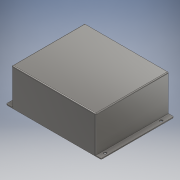
# Autodesk Inventor part: BatteryBox_NP1812
Saved by Autodesk Inventor 2018 (Build 220112000, 112)
## iProperties
Created: 2017-12-05
Part Number: BatteryBox_NP1812
Material: Steel, Galvanized
Document SubType Name: Modeling
Designer: P136265
Density: 7.85 g/cm^3
Appearance: Galvanized
Author: P136265
Autodesk Inventor part; units mm, degrees
ref_plane "YZ Plane" through (0, 0, 0) normal (1, 0, 0) x (0, 1, 0)
ref_plane "XZ Plane" through (0, 0, 0) normal (0, 1, 0) x (-1, 0, 0)
ref_plane "XY Plane" through (0, 0, 0) normal (0, 0, 1) x (1, 0, 0)
sketch "Sketch1" plane through (0, 0, 0) normal (0, 0, 1) x (1, 0, 0)
  line L0 (-92, -80) -> (92, -80)
  line L1 (92, -80) -> (92, 80)
  line L2 (92, 80) -> (-92, 80) construction
  line L3 (-92, 80) -> (-92, -80)
  line L4 (-92, -80) -> (92, 80) construction
  line L5 (92, -80) -> (-92, 80) construction
  line L6 (-92, -80) -> (-94, -80) construction
  line L7 (-92, 80) -> (-94, 80) construction
  line L8 (-92, -80) -> (-92, -82) construction
  line L9 (-94, 80) -> (-94, -82)
  line L10 (92, -80) -> (94, -80) construction
  line L11 (92, -80) -> (92, -82) construction
  line L12 (92, 80) -> (94, 80) construction
  line L13 (94, 80) -> (94, -82)
  line L14 (94, -82) -> (-94, -82)
  line L15 (-94, 80) -> (-92, 80)
  line L16 (92, 80) -> (94, 80)
  point P0 (0, 0)
  dimension "d0" = 184
  dimension "d1" = 160
  dimension "d2" = 2
  dimension "d3" = 2
  dimension "d4" = 2
  dimension "d5" = 2
  dimension "d6" = 2
  dimension "d7" = 2
  dimension "d8" = 2
  constraints: 34 end point, 4 perpendicular, 3 horizontal, 3 parallel, 2 midpoint, 2 point on line, 2 vertical, 1 collinear
  measures "d0" distance of L2.end L1.end
  measures "d1" distance of L1.end L0.end
  measures "d2" distance of L0.start L6.end
  measures "d3" distance of L2.end L7.end
  measures "d4" distance of L0.start L8.end
  measures "d5" distance of L0.end L10.end
  measures "d6" distance of L0.end L11.end
  measures "d7" distance of L1.end L12.end
  measures "d8" distance between parallel lines of L14 L0
extrude "Extrusion1" add sketch "Sketch1" along normal blind 80
sketch "Sketch2" plane through (0, 0, 80) normal (0, 0, 1) x (1, 0, 0)
  line L0 (92, -80) -> (-92, -80) construction
  line L1 (-92, -80) -> (-92, 80) construction
  line L2 (-92, 80) -> (-94, 80) construction
  line L3 (-94, 80) -> (-94, -82) construction
  line L4 (-94, -82) -> (94, -82) construction
  line L5 (94, -82) -> (94, 80) construction
  line L6 (94, 80) -> (92, 80) construction
  line L7 (92, 80) -> (92, -80) construction
  line L8 (-94, -82) -> (-94, 80) projected
  line L9 (94, -82) -> (94, 80) projected
  line L10 (-94, 80) -> (94, 80)
  line L11 (94, 80) -> (94, -82)
  line L12 (94, -82) -> (-94, -82)
  line L13 (-94, -82) -> (-94, 80)
  point P0 (0, 0)
  constraints: 8 end point, 2 parallel, 1 horizontal, 1 perpendicular
extrude "Extrusion2" add sketch "Sketch2" along normal blind 2
sketch "Sketch3" plane through (-94, -82, 0) normal (-1, 0, 0) x (0, 0, 1)
  line L0 (0, 0) -> (0, 162) construction
  line L1 (0, 0) -> (82, 0) construction
  line L2 (82, 162) -> (82, 0) construction
  line L3 (0, 162) -> (82, 162) construction
  line L4 (0, 162) -> (80, 162) construction
  line L5 (0, 0) -> (2, 0)
  line L6 (2, 0) -> (2, 162)
  line L7 (2, 162) -> (0, 162)
  line L8 (0, 162) -> (0, 0)
  point P0 (0, 82)
  dimension "d13" = 2
  constraints: 8 end point, 2 parallel, 1 horizontal, 1 perpendicular, 1 point on line
  measures "d13" distance of L7.end L6.end
extrude "Extrusion3" add sketch "Sketch3" along normal blind 12
sketch "Sketch4" plane through (94, -82, 0) normal (1, 0, 0) x (0, 0, -1)
  line L0 (0, 162) -> (0, 0) construction
  line L1 (0, 162) -> (-82, 162) construction
  line L2 (-82, 0) -> (-82, 162) construction
  line L3 (0, 0) -> (-82, 0) construction
  line L4 (0, 162) -> (0, 2) projected
  line L5 (-2, 0) -> (-82, 0) construction
  line L6 (0, 162) -> (-2, 162)
  line L7 (-2, 162) -> (-2, 0)
  line L8 (-2, 0) -> (0, 0)
  line L9 (0, 0) -> (0, 162)
  point P0 (0, 82)
  constraints: 8 end point, 2 parallel, 1 horizontal, 1 perpendicular
extrude "Extrusion4" add sketch "Sketch4" along normal blind 12
sketch "Sketch5" plane through (-94, -82, 2) normal (0, 0, 1) x (1, 0, 0)
  circle A0 centre (-6, 15) radius 3 construction
  line L0 (0, 162) -> (0, 0) construction
  line L1 (0, 162) -> (-12, 162) construction
  line L2 (-12, 0) -> (-12, 162) construction
  line L3 (0, 0) -> (-12, 0) construction
  circle A1 centre (-6, 140) radius 3 construction
  line L4 (188, 162) -> (0, 162) construction
  line L5 (0, 162) -> (0, 0) construction
  line L6 (0, 0) -> (188, 0) construction
  line L7 (188, 0) -> (188, 162) construction
  line L8 (188, 162) -> (0, 162) construction
  line L9 (94, 162) -> (94, 2) construction
  line L10 (2, 2) -> (186, 2) construction
  circle A2 centre (194, 15) radius 3 construction
  circle A3 centre (194, 140) radius 3 construction
  point P0 (94, 82)
  dimension "d18" = 6
  dimension "d19" = 15
  dimension "d23" = 6
  dimension "d24" = 125
  dimension "d25" = 100
  constraints: 4 centre point, 2 end point, 2 midpoint, 2 symmetric about line, 1 vertical alignment, 2 other
  measures "d18" diameter of A0
  measures "d19" distance from line of L3 A0.centre
  measures "d23" diameter of A1
  measures "d24" distance of A0.centre A1.centre
  measures "d25" distance from line of L9 A0.centre
hole "Hole1" at (-100, 58, 2) at (-100, -67, 2) at (100, -67, 2) at (100, 58, 2) direction (0, 0, -1) diameter 6 end through all
fillet "Fillet1" radius 2 9 edges at (-106, 80, 1) (-106, -82, 1) (106, -82, 1) (106, 80, 1) (94, -1, 82) (-94, -1, 82) (-94, -82, 42) (94, -82, 42) (0, -82, 82)
fillet "Fillet1" radius 0.25 6 edges at (0, 80, 80) (92, 80, 40) (-92, 80, 40) (-94, 80, 42) (0, 80, 82) (94, 80, 42)
body "Solid1"
